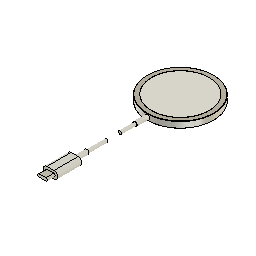
MagSafe_to_AMPS_adapter_v14 (Autodesk Fusion 360 archive; units mm, degrees)
design "MagSafe Chager"
Autodesk Fusion 360 part; units mm, degrees
sketch "Sketch1" plane through (0, 0, 0) normal (0, 0, 1) x (1, 0, 0) in component "Puck"
  circle A0 centre (0, 0) radius 27.94
  circle A1 centre (0, 0) radius 24.13
  dimension "d1" = 55.88
  dimension "d4" = 48.26
  constraint coincident A0.centre A1.centre
  measures "d1" diameter of A0
  measures "d4" diameter of A1
extrude "Extrude1" add sketch "Sketch1" along normal blind 5.2705 contours A0 | A1 makes body 1 in component "Puck"
extrude "Extrude2" add sketch "Sketch1" along normal blind 5.4102 contours A1 bodies 1 in component "Puck"
fillet "Fillet1" radius 0.254 2 edges at (-26.0492, -10.1035, 5.2705) (-26.0492, -10.1035, 0) on bodies 1 in component "Puck"
ref_plane "WorkPlane1" through (0, -27.94, 1.9338) normal (0, -1, 0) x (-1, 0, 0) in component "Puck"
sketch "Sketch2" plane through (0, -27.94, 1.9338) normal (0, -1, 0) x (1, 0, 0) in component "Puck"
  line L0 (27.94, 3.0827) -> (-27.94, 3.0827) construction
  line L1 (0, 3.0827) -> (0, -1.6798) construction
  line L2 (-27.94, -1.6798) -> (27.94, -1.6798) construction
  circle A0 centre (0, 0.7014) radius 1.905
  circle A1 centre (0, 0.7014) radius 1.3462
  dimension "d9" = 3.81
  dimension "d10" = 2.6924
  constraint midpoint L0 L1.start
  constraint perpendicular L0 L1
  constraint coincident L1.end L2
  constraint coincident L1 A0.centre
  constraint midpoint L1 A0.centre
  constraint concentric A0 A1
  measures "d9" diameter of A0
  measures "d10" diameter of A1
extrude "Extrude3" add sketch "Sketch2" along normal blind 10.16 and the other way blind 0.508 bodies 1 in component "Puck"
extrude "Extrude4" add sketch "Sketch2" along normal blind 22.86 and the other way blind 0.254 contours A1 bodies 1 in component "Puck"
sketch "Sketch1 (2)" plane through (0, 0, 0) normal (0, 1, 0) x (1, 0, 0) in component "USBC"
  line L0 (-6.1214, 0) -> (6.1214, 0) construction
  line L1 (-2.9718, -3.1496) -> (2.9718, -3.1496)
  arc A0 (2.9718, -3.1496) -> (2.9718, 3.1496) centre (2.9718, 0) ccw
  line L2 (2.9718, 3.1496) -> (-2.9718, 3.1496)
  arc A1 (-2.9718, 3.1496) -> (-2.9718, -3.1496) centre (-2.9718, 0) ccw
  line L3 (-6.1214, 0) -> (6.1214, 0) construction
  line L4 (-4.1021, 0) -> (4.1021, 0) construction
  line L5 (-2.9274, -1.1747) -> (2.9274, -1.1747)
  arc A2 (2.9274, -1.1747) -> (2.9274, 1.1747) centre (2.9274, 0) ccw
  line L6 (2.9274, 1.1747) -> (-2.9274, 1.1747)
  arc A3 (-2.9274, 1.1747) -> (-2.9274, -1.1747) centre (-2.9274, 0) ccw
  line L7 (-4.1021, 0) -> (4.1021, 0) construction
  circle A4 centre (0, 0) radius 1.8796
  circle A5 centre (0, 0) radius 1.3462
  dimension "d19" = 12.2428
  dimension "d20" = 6.2992
  dimension "d21" = 8.2042
  dimension "d22" = 2.3495
  dimension "d23" = 3.7592
  dimension "d24" = 2.6924
  constraint horizontal L0
  constraint midpoint A4.centre L0
  constraint tangent L1 A0
  constraint tangent A0 L2
  constraint parallel L1 L2
  constraint tangent L2 A1
  constraint tangent L1 A1
  constraint midpoint L0.start A1
  constraint midpoint L0.end A0
  constraint parallel L0 L3
  constraint parallel L3 L4
  constraint midpoint A4.centre L4
  constraint tangent L5 A2
  constraint tangent A2 L6
  constraint parallel L5 L6
  constraint tangent L6 A3
  constraint tangent L5 A3
  constraint midpoint L4.start A3
  constraint midpoint L4.end A2
  constraint coincident A4.centre A5.centre
  measures "d19" distance of L0.start L0.end
  measures "d20" diameter of A0
  measures "d21" distance of L4.start L4.end
  measures "d22" diameter of A2
  measures "d23" diameter of A4
  measures "d24" diameter of A5
extrude "Extrude1'" add sketch "Sketch1 (2)" along normal blind 20.447 separate body contours L1 A0 L2 A1 | L5 A4 A5 | L5 A5 | L6 A4 A5 | L6 A5 makes body 2 in component "USBC"
extrude "Extrude2'" add sketch "Sketch1 (2)" along normal blind 27.1399 contours L5 L6 A3 A4 | L5 L6 A4 A5 | L5 L6 A5 | L5 A2 L6 A4 | L5 L6 A4 A5 bodies 2 in component "USBC"
extrude "Extrude3'" add sketch "Sketch1 (2)" against normal blind 10.16 contours L5 L6 A4 A5 | L5 A4 A5 | L6 A4 A5 | L5 L6 A4 A5 bodies 2 in component "USBC"
extrude "Extrude4'" add sketch "Sketch1 (2)" against normal blind 26.67 contours L5 L6 A5 | L5 A5 | L6 A5 bodies 2 in component "USBC"
component "Puck" placed x (1, 0, 0) y (0, 1, 0) z (0, 0, 1) at (0, 0, 0)
component "USBC" placed x (-1, 0, 0) y (0, -1, 0) z (0, 0, 1) at (0, -88.9, 2.6353)
equation "d1 = 2.2 \""
equation "d2 = 0.2075 \""
equation "d4 = 1.9 \""
equation "d5 = 0.213 \""
equation "d7 = 0.01 \""
equation "d9 = 0.15 \""
equation "d10 = 0.106 \""
equation "d11 = 0.4 \""
equation "d13 = 0.02 \""
equation "d14 = 0.0 °"
equation "d15 = 0.90 \""
equation "d17 = 0.01 \""
equation "d18 = 0.0 °"
equation "d19 = 0.482 \""
equation "d20 = 0.248 \""
equation "d21 = 0.323 \""
equation "d22 = 0.0925 \""
equation "d23 = 0.148 \""
equation "d24 = 0.106 \""
equation "d25 = 0.805 \""
equation "d27 = 1.0685 \""
equation "d29 = -0.4 \""
equation "d31 = -1.05 \""

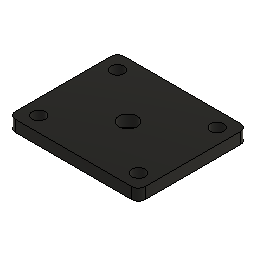
design "Tilt Swivel AMPS Proclip:215500"
Autodesk Fusion 360 part; units mm, degrees
sketch "Sketch1" plane through (0, 0, 0) normal (0, 0, 1) x (1, 0, 0)
  line L0 (-19, 15) -> (19, 15) construction
  line L1 (19, 15) -> (19, -15) construction
  line L2 (19, -15) -> (-19, -15) construction
  line L3 (-19, -15) -> (-19, 15) construction
  line L4 (-19, 15) -> (19, -15) construction
  line L5 (-22.1996, 20.7518) -> (22.1996, 20.7518)
  line L6 (24.7396, 18.2118) -> (24.7396, -18.2118)
  line L7 (22.1996, -20.7518) -> (-22.1996, -20.7518)
  line L8 (-24.7396, -18.2118) -> (-24.7396, 18.2118)
  circle A0 centre (19, 15) radius 2.5
  circle A1 centre (19, -15) radius 2.5
  circle A2 centre (-19, -15) radius 2.5
  circle A3 centre (-19, 15) radius 2.5
  line L9 (-24.7396, 20.7518) -> (24.7396, -20.7518) construction
  arc A4 (-24.7396, -18.2118) -> (-22.1996, -20.7518) centre (-22.1996, -18.2118) ccw
  arc A5 (-22.1996, 20.7518) -> (-24.7396, 18.2118) centre (-22.1996, 18.2118) ccw
  arc A6 (24.7396, 18.2118) -> (22.1996, 20.7518) centre (22.1996, 18.2118) ccw
  arc A7 (22.1996, -20.7518) -> (24.7396, -18.2118) centre (22.1996, -18.2118) ccw
  circle A8 centre (0, 0) radius 3.4925
  point P0 (24.7396, 20.7518)
  point P1 (-24.7396, -20.7518)
  dimension "d1" = 38
  dimension "d2" = 30
  dimension "d3" = 48.4149
  dimension "d4" = 5
  dimension "d5" = 41.5036
  dimension "d6" = 49.4792
  dimension "d7" = 2.54
  dimension "d8" = 2.54
  dimension "d9" = 2.54
  dimension "d10" = 2.54
  dimension "d14" = 6.985
  constraint horizontal L0
  constraint vertical L1
  constraint horizontal L2
  constraint vertical L3
  constraint midpoint A8.centre L4
  constraint horizontal L5
  constraint vertical L6
  constraint horizontal L7
  constraint vertical L8
  constraint coincident L0.end L1.start
  constraint coincident L1.end L2.start
  constraint coincident L2.end L3.start
  constraint coincident L0.start L3.end
  constraint equal A2 A3
  constraint equal A1 A2
  constraint equal A0 A1
  constraint midpoint A8.centre L9
  constraint coincident P1 L7
  constraint coincident P1 L8
  constraint tangent L7 A4
  constraint tangent L8 A4
  constraint coincident L9.start L5
  constraint coincident L9.start L8
  constraint tangent L5 A5
  constraint tangent L8 A5
  constraint coincident P0 L5
  constraint coincident P0 L6
  constraint tangent L5 A6
  constraint tangent L6 A6
  constraint coincident L9.end L6
  constraint coincident L9.end L7
  constraint tangent L6 A7
  constraint tangent L7 A7
  constraint coincident A8.centre origin
  measures "d1" distance of L0.start L0.end
  measures "d2" distance of L0.start L2.end
  measures "d3" distance of L0.start L1.end
  measures "d4" diameter of A0
  measures "d5" distance of P0 L9.end
  measures "d6" distance of L9.end P1
  measures "d7" radius of A4
  measures "d8" radius of A5
  measures "d9" radius of A6
  measures "d10" radius of A7
  measures "d14" diameter of A8
extrude "Extrude1" add sketch "Sketch1" along normal blind 4.318
sketch "Sketch2" plane through (0, 0, 0) normal (0, 0, -1) x (1, 0, 0)
  circle A0 centre (-19, 15) radius 2.5
  circle A1 centre (19, -15) radius 2.5
  circle A2 centre (-19, -15) radius 2.5
  circle A3 centre (19, 15) radius 2.5
  arc A4 (-22.1996, 20.7518) -> (-24.7396, 18.2118) centre (-22.1996, 18.2118) ccw
  line L0 (-24.7396, 18.2118) -> (-24.7396, -18.2118)
  arc A5 (-24.7396, -18.2118) -> (-22.1996, -20.7518) centre (-22.1996, -18.2118) ccw
  line L1 (-22.1996, -20.7518) -> (22.1996, -20.7518)
  arc A6 (22.1996, -20.7518) -> (24.7396, -18.2118) centre (22.1996, -18.2118) ccw
  line L2 (24.7396, -18.2118) -> (24.7396, 18.2118)
  arc A7 (24.7396, 18.2118) -> (22.1996, 20.7518) centre (22.1996, 18.2118) ccw
  line L3 (22.1996, 20.7518) -> (-22.1996, 20.7518)
  circle A8 centre (0, 0) radius 16.891
  circle A9 centre (0, 0) radius 3.4925
  dimension "d13" = 33.782
  constraint coincident A8.centre A9.centre
  measures "d13" diameter of A8
equation "d3 = 1.906097 \""
equation "d5 = 1.634 \""
equation "d6 = 1.948 \""
equation "d7 = 0.10 \""
equation "d8 = 0.1 \""
equation "d9 = 0.1 \""
equation "d10 = 0.1 \""
equation "d11 = 0.17 \""
equation "d13 = 1.33 \""
equation "d14 = 0.275 \""
